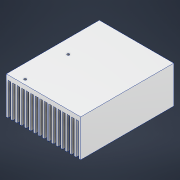
# Autodesk Inventor part: heatsink
Saved by Autodesk Inventor 2022 (Build 260153000, 153)
## iProperties
Created: 2023-06-09
Part Number: heatsink
Material: Aluminum 6061
Document SubType Name: Modeling
Designer: voids
Density: 2.7 g/cm^3
Appearance: Aluminum - Flat
Author: voids
Autodesk Inventor part; units mm, degrees
ref_plane "YZ Plane" through (0, 0, 0) normal (1, 0, 0) x (0, 1, 0)
ref_plane "XZ Plane" through (0, 0, 0) normal (0, 1, 0) x (-1, 0, 0)
ref_plane "XY Plane" through (0, 0, 0) normal (0, 0, 1) x (1, 0, 0)
sketch "Sketch1" plane through (0, 0, 0) normal (0, 0, 1) x (1, 0, 0)
  line L0 (0, 0) -> (80, 0)
  line L1 (80, 0) -> (80, 40)
  line L2 (80, 40) -> (0, 40)
  line L3 (0, 40) -> (0, 0)
  line L4 (2, 0) -> (4.875, 0)
  line L5 (4.875, 0) -> (4.875, 35)
  line L6 (4.875, 35) -> (2, 35)
  line L7 (2, 35) -> (2, 0)
  line L8 (6.875, 35) -> (6.875, 0)
  line L9 (9.75, 35) -> (6.875, 35)
  line L10 (6.875, 0) -> (9.75, 0)
  line L11 (9.75, 0) -> (9.75, 35)
  line L12 (11.75, 35) -> (11.75, 0)
  line L13 (14.625, 35) -> (11.75, 35)
  line L14 (11.75, 0) -> (14.625, 0)
  line L15 (14.625, 0) -> (14.625, 35)
  line L16 (16.625, 35) -> (16.625, 0)
  line L17 (19.5, 35) -> (16.625, 35)
  line L18 (16.625, 0) -> (19.5, 0)
  line L19 (19.5, 0) -> (19.5, 35)
  line L20 (21.5, 35) -> (21.5, 0)
  line L21 (24.375, 35) -> (21.5, 35)
  line L22 (21.5, 0) -> (24.375, 0)
  line L23 (24.375, 0) -> (24.375, 35)
  line L24 (26.375, 35) -> (26.375, 0)
  line L25 (29.25, 35) -> (26.375, 35)
  line L26 (26.375, 0) -> (29.25, 0)
  line L27 (29.25, 0) -> (29.25, 35)
  line L28 (31.25, 35) -> (31.25, 0)
  line L29 (34.125, 35) -> (31.25, 35)
  line L30 (31.25, 0) -> (34.125, 0)
  line L31 (34.125, 0) -> (34.125, 35)
  line L32 (36.125, 35) -> (36.125, 0)
  line L33 (39, 35) -> (36.125, 35)
  line L34 (36.125, 0) -> (39, 0)
  line L35 (39, 0) -> (39, 35)
  line L36 (41, 35) -> (41, 0)
  line L37 (43.875, 35) -> (41, 35)
  line L38 (41, 0) -> (43.875, 0)
  line L39 (43.875, 0) -> (43.875, 35)
  line L40 (45.875, 35) -> (45.875, 0)
  line L41 (48.75, 35) -> (45.875, 35)
  line L42 (45.875, 0) -> (48.75, 0)
  line L43 (48.75, 0) -> (48.75, 35)
  line L44 (50.75, 35) -> (50.75, 0)
  line L45 (53.625, 35) -> (50.75, 35)
  line L46 (50.75, 0) -> (53.625, 0)
  line L47 (53.625, 0) -> (53.625, 35)
  line L48 (55.625, 35) -> (55.625, 0)
  line L49 (58.5, 35) -> (55.625, 35)
  line L50 (55.625, 0) -> (58.5, 0)
  line L51 (58.5, 0) -> (58.5, 35)
  line L52 (60.5, 35) -> (60.5, 0)
  line L53 (63.375, 35) -> (60.5, 35)
  line L54 (60.5, 0) -> (63.375, 0)
  line L55 (63.375, 0) -> (63.375, 35)
  line L56 (65.375, 35) -> (65.375, 0)
  line L57 (68.25, 35) -> (65.375, 35)
  line L58 (65.375, 0) -> (68.25, 0)
  line L59 (68.25, 0) -> (68.25, 35)
  line L60 (70.25, 35) -> (70.25, 0)
  line L61 (73.125, 35) -> (70.25, 35)
  line L62 (70.25, 0) -> (73.125, 0)
  line L63 (73.125, 0) -> (73.125, 35)
  line L64 (75.125, 35) -> (75.125, 0)
  line L65 (78, 35) -> (75.125, 35)
  line L66 (75.125, 0) -> (78, 0)
  line L67 (78, 0) -> (78, 35)
  dimension "d0" = 40
  dimension "d1" = 80
  dimension "d2" = 2
  dimension "d3" = 5
  dimension "d6" = 4.875
  dimension "d11" = 2
  dimension "d12" = 2
  constraints: 134 end point, 3 horizontal, 3 parallel, 1 perpendicular, 1 vertical, 124 other
  measures "d0" distance of L1.end L1.start
  measures "d1" distance of L1.end L2.end
  measures "d2" distance between parallel lines of L3 L7
  measures "d3" distance between parallel lines of L2 L6
  measures "d6" distance of L6.end L8.start
  measures "d11" distance between parallel lines of L1 L67
  measures "d12" distance between parallel lines of L8 L5
extrude "Extrusion1" add sketch "Sketch1" along normal blind 100 contours L3 L2 L1 L0 L67 L65 L64 L63 L61 L60 L59 L57 L56 L55 L53 L52 L51 L49 L48 L47 L45 L44 L43 L41 L40 L39 L37 L36 L35 L33 L32 L31 L29 L28 L27 L25 L24 L23 L21 L20 L19 L17 L16 L15 L13 L12 L11 L9 L8 L5 L6 L7
sketch "Sketch2" plane through (0, 40, 0) normal (0, 1, 0) x (1, 0, 0)
  line L0 (15.24, -94.8438) -> (15.24, -48.6158) construction
  line L1 (4.875, 0) -> (4.875, -100) construction
  line L2 (0, 0) -> (0, -100) construction
  line L3 (80, -100) -> (0, -100) construction
  dimension "d15" = 46.228
  dimension "d17" = 15.24
  dimension "d18" = 5.1562
  constraints: 2 coincident, 2 end point, 1 vertical
  measures "d15" distance of L0.start L0.end
  measures "d17" distance between parallel lines of L2 L0
  measures "d18" distance from line of L3 L0.start
hole "Hole1" at (15.24, 40, 94.8438) at (15.24, 40, 48.6158) direction (0, -1, 0) diameter 2.459 depth 5 tip angle 118 start extended yes thread size "M3x0.5" class "6H" standard "ANSI Metric M Profile"
equation "\"d11\" = d2"
equation "\"d12\" = d2"
body "Solid1"
